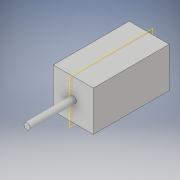
# Autodesk Inventor part: Square-Circle-Adapter V1D2-OUT
Saved by Autodesk Inventor 2017 (Build 210142000, 142)
## iProperties
Created: 2017-12-22
Part Number: Square-Circle-Adapter V1D2-OUT
Material: Generic
Document SubType Name: Modeling
Designer: Tripl_000
Density: 1 g/cm^3
Appearance: Default
Author: Tripl_000
Autodesk Inventor part; units mm, degrees
ref_plane "YZ Plane" through (0, 0, 0) normal (1, 0, 0) x (0, 1, 0)
ref_plane "XZ Plane" through (0, 0, 0) normal (0, 1, 0) x (-1, 0, 0)
ref_plane "XY Plane" through (0, 0, 0) normal (0, 0, 1) x (1, 0, 0)
sketch "Sketch1" plane through (0, 0, 0) normal (0, 0, 1) x (1, 0, 0)
  line L0 (-6.604, 6.604) -> (6.604, 6.604)
  line L1 (6.604, 6.604) -> (6.604, -6.604)
  line L2 (6.604, -6.604) -> (-6.604, -6.604)
  line L3 (-6.604, -6.604) -> (-6.604, 6.604)
  line L4 (-6.604, 6.604) -> (6.604, -6.604) construction
  line L5 (6.604, 6.604) -> (-6.604, -6.604) construction
  point P0 (0, 0)
  dimension "d0" = 13.208
  dimension "d1" = 13.208
  constraints: 12 end point, 2 midpoint, 2 parallel, 1 horizontal, 1 perpendicular
  measures "d0" distance of L2.end L0.start
  measures "d1" distance of L0.start L0.end
extrude "Extrusion1" add sketch "Sketch1" along normal blind 15
sketch "Sketch2" plane through (0, 0, 15) normal (0, 0, 1) x (1, 0, 0)
  line L0 (-5.0165, 5.0165) -> (5.0165, 5.0165)
  line L1 (5.0165, 5.0165) -> (5.0165, -5.0165)
  line L2 (5.0165, -5.0165) -> (-5.0165, -5.0165)
  line L3 (-5.0165, -5.0165) -> (-5.0165, 5.0165)
  line L4 (-5.0165, 5.0165) -> (5.0165, -5.0165) construction
  line L5 (5.0165, 5.0165) -> (-5.0165, -5.0165) construction
  point P0 (0, 0)
  dimension "d4" = 10.033
  dimension "d5" = 10.033
  constraints: 12 end point, 2 midpoint, 2 parallel, 1 horizontal, 1 perpendicular
  measures "d4" distance of L0.end L1.end
  measures "d5" distance of L0.start L0.end
extrude "Extrusion2" cut sketch "Sketch2" against normal through all
sketch "Sketch5" plane through (0, 0, 15) normal (0, 0, 1) x (1, 0, 0)
  line L0 (6.604, 6.604) -> (-6.604, 6.604) projected
  line L1 (6.604, 6.604) -> (6.604, -6.604) projected
  line L2 (-6.604, 6.604) -> (6.604, 6.604)
  line L3 (6.604, 6.604) -> (6.604, -6.604)
  line L4 (6.604, -6.604) -> (-6.604, -6.604)
  line L5 (-6.604, -6.604) -> (-6.604, 6.604)
  point P0 (0, 0)
  constraints: 8 end point, 2 parallel, 1 horizontal, 1 perpendicular
extrude "Extrusion5" add sketch "Sketch5" along normal blind 10
sketch "Sketch8" plane through (0, 0, 25) normal (0, 0, 1) x (1, 0, 0)
  circle A0 centre (0, 0) radius 0.762
  dimension "d44" = 1.524
  constraints: 1 centre point, 1 coincident
  measures "d44" diameter of A0
extrude "Extrusion7" add sketch "Sketch8" along normal blind 15.24
sketch "Sketch9" plane through (0, 0, 25) normal (0, 0, 1) x (1, 0, 0)
  circle A0 centre (0, 0) radius 1.016
  dimension "d47" = 2.032
  constraints: 1 centre point, 1 coincident
  measures "d47" diameter of A0
extrude "Extrusion8" add sketch "Sketch9" along normal up to surface (15.24 mm away)
ref_plane "Work Plane3" through (0, -6.604, 0) normal (1, 0, 0) x (0, 0, -1)
body "Solid1"
